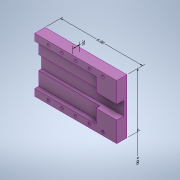
# Autodesk Inventor part: pistonHousing
Saved by Autodesk Inventor 2020.2 (Build 242310000, 310)
## iProperties
Created: 2020-01-13
Part Number: pistonHousing
Material: PET Plastic
Document SubType Name: Modeling
Designer: robst
Density: 1.541 g/cm^3
Appearance: Smooth - Purple
Author: robst
Autodesk Inventor part; units mm, degrees
ref_plane "YZ Plane" through (0, 0, 0) normal (1, 0, 0) x (0, 1, 0)
ref_plane "XZ Plane" through (0, 0, 0) normal (0, 1, 0) x (-1, 0, 0)
sketch "Sketch1" plane through (0, 0, 0) normal (0, 0, 1) x (1, 0, 0)
  line L0 (-76.2, -50.8) -> (76.2, -50.8)
  line L1 (76.2, -50.8) -> (76.2, 50.8)
  line L2 (76.2, 50.8) -> (-76.2, 50.8)
  line L3 (-76.2, 50.8) -> (-76.2, -50.8)
  line L4 (-76.2, -50.8) -> (76.2, 50.8) construction
  line L5 (76.2, -50.8) -> (-76.2, 50.8) construction
  point P0 (0, 0)
  dimension "d0" = 152.4
  dimension "d1" = 101.6
  constraints: 12 end point, 2 midpoint, 2 parallel, 1 horizontal, 1 perpendicular
  measures "d0" distance of L2.end L1.end
  measures "d1" distance of L1.end L0.end
extrude "Extrusion1" add sketch "Sketch1" along normal mid plane 19.05
sketch "Sketch3" plane through (0, 0, 9.525) normal (0, 0, 1) x (1, 0, 0)
  line L0 (-76.2, -12.7) -> (76.2, -12.7)
  line L1 (76.2, -12.7) -> (76.2, 12.7)
  line L2 (76.2, 12.7) -> (-76.2, 12.7)
  line L3 (-76.2, 12.7) -> (-76.2, -12.7)
  line L4 (-76.2, -12.7) -> (76.2, 12.7) construction
  line L5 (76.2, -12.7) -> (-76.2, 12.7) construction
  point P0 (0, 0)
  dimension "d7" = 25.4
  dimension "d19" = 152.4
  constraints: 12 end point, 2 midpoint, 2 parallel, 1 horizontal, 1 perpendicular
  measures "d7" distance of L1.end L0.end
  measures "d19" distance of L1.end L2.end
extrude "Extrusion3" cut sketch "Sketch3" against normal blind 12.7
ref_plane "Work Plane1" through (-76.2, 50.8, 9.525) normal (0, 0, 1) x (1, 0, 0)
sketch "Sketch8" plane through (0, 0, 9.525) normal (0, 0, 1) x (1, 0, 0)
  line L0 (-76.2, -12.7) -> (-76.2, 12.7) projected
  line L1 (-76.2, 0) -> (38.1, 0)
  line L2 (38.1, 0) -> (38.1, 38.1)
  line L3 (38.1, 38.1) -> (-76.2, 38.1)
  line L4 (-76.2, 38.1) -> (-76.2, 0)
  line L5 (38.1, 0) -> (38.1, -38.1)
  line L6 (38.1, -38.1) -> (-76.2, -38.1)
  line L7 (-76.2, -38.1) -> (-76.2, 0)
  point P0 (0, 0)
  dimension "d51" = 114.3
  dimension "d52" = 38.1
  constraints: 14 end point, 2 parallel, 2 symmetric about line, 1 horizontal, 1 midpoint, 1 perpendicular
  measures "d51" distance of L3.end L2.end
  measures "d52" distance of L2.end L1.end
extrude "Extrusion6" cut sketch "Sketch8" against normal blind 7.366
sketch "Sketch9" plane through (0, 0, 9.525) normal (0, 0, 1) x (1, 0, 0)
  line L0 (-76.2, 50.8) -> (-76.2, 38.1) construction
  line L1 (-76.2, 44.45) -> (76.2, 44.45) construction
  line L2 (76.2, 50.8) -> (76.2, -50.8) construction
  line L3 (-76.2, 44.45) -> (-76.2, -44.4609) construction
  point P0 (0, 0)
  point P1 (-50.8, 44.45)
  point P2 (-25.4, 44.45)
  point P3 (0, 44.45)
  point P4 (25.4, 44.45)
  point P5 (50.8, 44.45)
  point P6 (-50.8, -44.45)
  point P7 (-25.4, -44.45)
  point P8 (0, -44.45)
  point P9 (25.4, -44.45)
  point P10 (50.8, -44.45)
  point P11 (-50.8, -133.35)
  point P12 (-25.4, -133.35)
  point P13 (0, -133.35)
  point P14 (25.4, -133.35)
  point P15 (50.8, -133.35)
  point P16 (-50.8, -222.25)
  point P17 (-25.4, -222.25)
  point P18 (0, -222.25)
  point P19 (25.4, -222.25)
  point P20 (50.8, -222.25)
  dimension "d55" = 25.4
  dimension "d58" = 25.4
  dimension "d61" = 88.9
  constraints: 4 end point, 2 horizontal, 2 point on line, 2 vertical, 1 midpoint, 19 other
  measures "d55" distance from line of L0 point (-50.8, 44.45)
  measures "d58" distance of point (-50.8, 44.45) point (-25.4, 44.45)
  measures "d61" distance of point (-50.8, 44.45) point (-50.8, -44.45)
hole "Hole2" at (-50.8, 44.45, 9.525) at (-25.4, 44.45, 9.525) at (0, 44.45, 9.525) at (25.4, 44.45, 9.525) at (50.8, 44.45, 9.525) at (-50.8, -44.45, 9.525) at (-25.4, -44.45, 9.525) at (0, -44.45, 9.525) at (25.4, -44.45, 9.525) at (50.8, -44.45, 9.525) at (-50.8, -133.35, 9.525) at (-25.4, -133.35, 9.525) at (0, -133.35, 9.525) at (25.4, -133.35, 9.525) at (50.8, -133.35, 9.525) at (-50.8, -222.25, 9.525) at (-25.4, -222.25, 9.525) at (0, -222.25, 9.525) at (25.4, -222.25, 9.525) at (50.8, -222.25, 9.525) direction (0, 0, -1) diameter 5.1054 end through all clearance for "Flat Head Machine Screw (82)" size "#10" standard "Ansi Unified Screw Threads"
body "Solid1"
